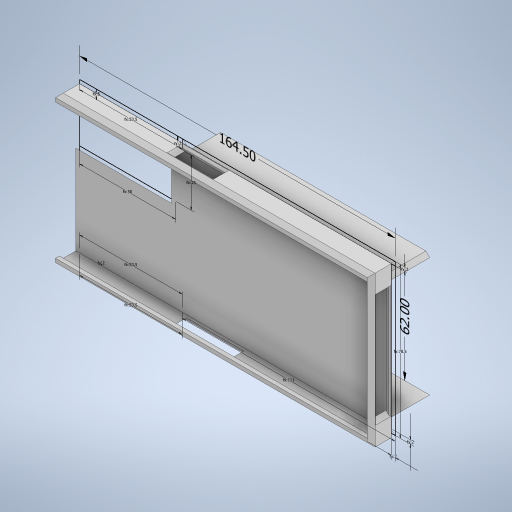
# Autodesk Inventor part: Case
Saved by Autodesk Inventor 2024 (Build 280153000, 153)
## iProperties
Created: 2024-07-02
Part Number: Case
Material: Generic
Document SubType Name: Modeling
Designer: Andrei
Density: 1 g/cm^3
Appearance: Default
Author: Andrei
Autodesk Inventor part; units mm, degrees
ref_plane "YZ Plane" through (0, 0, 0) normal (1, 0, 0) x (0, 1, 0)
ref_plane "XZ Plane" through (0, 0, 0) normal (0, 1, 0) x (-1, 0, 0)
ref_plane "XY Plane" through (0, 0, 0) normal (0, 0, 1) x (1, 0, 0)
sketch "Sketch1" plane through (0, 0, 0) normal (0, 0, 1) x (1, 0, 0)
  line L0 (-55.5, 39.25) -> (55.5, 39.25)
  line L1 (55.5, 39.25) -> (55.5, -39.25)
  line L2 (55.5, -39.25) -> (-55.5, -39.25)
  line L3 (-55.5, -39.25) -> (-55.5, 39.25)
  line L4 (-55.5, 39.25) -> (55.5, -39.25) construction
  line L5 (55.5, 39.25) -> (-55.5, -39.25) construction
  line L6 (-55.5, 39.25) -> (55.5, 39.25)
  line L7 (55.5, 39.25) -> (55.5, 37.25)
  line L8 (55.5, 37.25) -> (-55.5, 37.25)
  line L9 (-55.5, 37.25) -> (-55.5, 39.25)
  line L10 (55.5, 37.25) -> (53.5, 37.25)
  line L11 (53.5, 37.25) -> (53.5, -39.25)
  line L12 (53.5, -39.25) -> (55.5, -39.25)
  line L13 (55.5, -39.25) -> (55.5, 37.25)
  line L14 (-55.5, -39.25) -> (53.5, -39.25)
  line L15 (53.5, -39.25) -> (53.5, -37.25)
  line L16 (53.5, -37.25) -> (-55.5, -37.25)
  line L17 (-55.5, -37.25) -> (-55.5, -39.25)
  line L18 (-55.5, 39.25) -> (-109, 39.25)
  line L19 (-109, 39.25) -> (-109, -39.25)
  line L20 (-109, -39.25) -> (-55.5, -39.25)
  line L21 (-55.5, -39.25) -> (-55.5, 39.25)
  line L22 (-109, 34.25) -> (-59, 34.25)
  line L23 (-59, 34.25) -> (-59, 9.25)
  line L24 (-59, 9.25) -> (-109, 9.25)
  line L25 (-109, 9.25) -> (-109, 34.25)
  line L26 (-55.5, 39.25) -> (-109, 39.25)
  line L27 (-109, 39.25) -> (-109, 37.25)
  line L28 (-109, 37.25) -> (-55.5, 37.25)
  line L29 (-55.5, 37.25) -> (-55.5, 39.25)
  line L30 (-55.5, -39.25) -> (-109, -39.25)
  line L31 (-109, -39.25) -> (-109, -37.25)
  line L32 (-109, -37.25) -> (-55.5, -37.25)
  line L33 (-55.5, -37.25) -> (-55.5, -39.25)
  point P0 (0, 0)
  point P1 (-55.5, -37.25)
  point P2 (-55.5, 37.25)
  point P3 (-55.5, -37.25)
  dimension "d0" = 111
  dimension "d1" = 78.5
  dimension "d2" = 2
  dimension "d3" = 2
  dimension "d4" = 2
  dimension "d5" = 53.5
  dimension "d80" = 50
  dimension "d81" = 25
  dimension "d82" = 5
  dimension "d91" = 53.5
  dimension "d92" = 2
  dimension "d93" = 53.5
  dimension "d94" = 2
  constraints: 68 end point, 16 parallel, 8 horizontal, 8 perpendicular, 4 point on line, 2 midpoint
  measures "d0" distance of L1.end L2.end
  measures "d1" distance of L0.end L1.end
  measures "d2" distance of L6.end L7.end
  measures "d3" distance of L12.end L11.end
  measures "d4" distance of L15.end L14.end
  measures "d5" distance of L20.end L19.end
  measures "d80" distance of L23.end L24.end
  measures "d81" distance of L22.end L23.end
  measures "d82" distance between parallel lines of L18 L22
  measures "d91" distance of L28.end L27.end
  measures "d92" distance between parallel lines of L18 L28
  measures "d93" distance of L31.end L32.end
  measures "d94" distance between parallel lines of L30 L32
extrude "Extrusion1" add sketch "Sketch1" along normal blind 2 contours L8 L11 L16 L3
extrude "Extrusion2" add sketch "Sketch1" along normal blind 12.5 contours L0 L1 L8 L3 | L1 L2 L11 L8 | L16 L11 L2 L3
chamfer "Chamfer1" distance 2 angle 45 1 edges at (0, 39.25, 0)
chamfer "Chamfer2" distance 2 angle 45 1 edges at (55.5, -1, 0)
chamfer "Chamfer3" distance 2 angle 45 1 edges at (-1, -39.25, 0)
chamfer "Chamfer9" distance 2 angle 45 1 edges at (55.5, 0, 12.5)
extrude "Extrusion3" add sketch "Sketch1" along normal blind 2 contours L3 L28 L19 L18 | L3 L32 L19 L24 L23 L22 L28 | L3 L20 L19 L32 | L22 L23 L24 L19
chamfer "Chamfer13" distance 2 angle 45 1 edges at (-82.25, 39.25, 0)
chamfer "Chamfer14" distance 2 angle 45 1 edges at (-109, -1, 0)
chamfer "Chamfer15" distance 2 angle 45 1 edges at (-81.25, -39.25, 0)
sketch "Sketch2" plane through (0, 0, 0) normal (0, 0, -1) x (-1, 0, 0)
  line L0 (-53.5, 32) -> (53.5, 32)
  line L1 (53.5, 32) -> (53.5, -32)
  line L2 (53.5, -32) -> (-53.5, -32)
  line L3 (-53.5, -32) -> (-53.5, 32)
  line L4 (-53.5, 32) -> (53.5, -32) construction
  line L5 (53.5, 32) -> (-53.5, -32) construction
  line L6 (-53.5, -37.25) -> (-53.5, 37.25) projected
  line L7 (-53.5, 32) -> (57.5, 32)
  line L8 (57.5, 32) -> (57.5, 30)
  line L9 (57.5, 30) -> (-53.5, 30)
  line L10 (-53.5, 30) -> (-53.5, 32)
  line L11 (-53.5, -32) -> (55.5, -32)
  line L12 (55.5, -32) -> (55.5, -35.2285)
  line L13 (-53.5, -35.2285) -> (-53.5, -32)
  line L14 (-53.5, -32) -> (57.5, -32)
  line L15 (57.5, -32) -> (57.5, -34)
  line L16 (57.5, -34) -> (-53.5, -34)
  line L17 (-53.5, -34) -> (-53.5, -32)
  line L18 (57.5, 30) -> (61.5, 30)
  line L19 (61.5, -32) -> (59.5, -32)
  line L20 (57.5, 30) -> (55.5, 30)
  line L21 (55.5, 30) -> (55.5, -32)
  line L22 (55.5, -32) -> (57.5, -32)
  line L23 (57.5, -32) -> (57.5, 30)
  point P0 (0, 0)
  point P1 (55.5, 30)
  point P2 (-53.5, -32)
  dimension "d57" = 107
  dimension "d58" = 64
  dimension "d59" = 111
  dimension "d60" = 2
  dimension "d61" = 109
  dimension "d62" = 111
  dimension "d63" = 2
  dimension "d64" = 2
  dimension "d65" = 2
  constraints: 46 end point, 10 parallel, 7 point on line, 6 horizontal, 5 perpendicular, 2 midpoint
  measures "d57" distance of L0.start L0.end
  measures "d58" distance of L0.end L1.end
  measures "d59" distance of L8.end L9.end
  measures "d60" distance of L7.end L8.end
  measures "d61" distance of L12.end L13.start
  measures "d62" distance of L15.end L16.end
  measures "d63" distance between parallel lines of L16 L14
  measures "d64" distance of L19.start L19.end
  measures "d65" distance of L22.end L21.end
extrude "Extrusion4" add sketch "Sketch2" along normal blind 20 contours L0 L1 L9 L3 | L7 L8 L9 L1 | L2 L11 L12 L16 L6 | L9 L23 L14 L21 | L14 L15 L16 L12
chamfer "Chamfer16" distance 2 angle 45 4 edges at (-57.5, -34, -10) (-57.5, 32, -10) (53.5, 32, -10) (53.5, -34, -10)
sketch "Sketch3" plane through (-57.5, -32, 0) normal (-1, 0, 0) x (0, 0, 1)
  line L0 (0, 0) -> (-20, 0) projected
  line L1 (0, 62) -> (-20, 62) projected
  line L2 (-20, 0) -> (0, 62)
  line L3 (-20, 62) -> (-20, 64) projected
  line L4 (-20, 62) -> (0, 0)
  circle A0 centre (-10, 31) radius 2.5
  point P0 (0, 32)
  dimension "d71" = 5
  constraints: 4 end point, 1 centre point, 1 midpoint
  measures "d71" diameter of A0
hole "Hole1" at (-57.5, -1, -10) direction (1, 0, 0) diameter 9.2964 end through all counterbore diameter 9.525 counterbore depth 5
extrude "Extrusion5" cut sketch "Sketch1" along normal blind 10 contours L22 L23 L24 L19
chamfer "Chamfer17" distance 1 angle 45 1 edges at (-59, 21.75, 0)
chamfer "Chamfer18" distance 2 angle 45 4 edges at (-58.5, 34.25, 0) (-83.0001, 34.25, 0) (-58.5, 9.25, 0) (-83.0001, 9.25, 0)
extrude "Extrusion6" add sketch "Sketch1" along normal blind 12.5 contours L3 L28 L19 L18 | L3 L20 L19 L32
chamfer "Chamfer19" distance 2 angle 45 6 edges at (-27.7499, -39.25, 12.5) (-27.75, 39.25, 12.5) (-109, -39.25, 6.25) (-109, 39.25, 6.25) (-82.25, 39.25, 0) (-82.25, -39.25, 0)
sketch "Sketch4" plane through (55.5, -39.25, 2) normal (1, 0, 0) x (0, 0, -1)
  line L0 (0, 0) -> (-8.5, 0) projected
  line L1 (0, 78.5) -> (0, 0) projected
  line L2 (-8.5, 0) -> (0, 78.5)
  line L3 (-8.5, 0) -> (-8.5, 78.5) projected
  line L4 (-8.5, 78.5) -> (0, 0)
  line L5 (-7.75, 11.75) -> (-0.75, 11.75)
  line L6 (-0.75, 11.75) -> (-0.75, 66.75)
  line L7 (-0.75, 66.75) -> (-7.75, 66.75)
  line L8 (-7.75, 66.75) -> (-7.75, 11.75)
  line L9 (-7.75, 11.75) -> (-0.75, 66.75) construction
  line L10 (-0.75, 11.75) -> (-7.75, 66.75) construction
  point P0 (2, 39.25)
  point P1 (-4.25, 39.25)
  dimension "d100" = 7
  dimension "d101" = 55
  constraints: 16 end point, 3 midpoint, 2 parallel, 1 horizontal, 1 perpendicular
  measures "d100" distance of L7.end L6.end
  measures "d101" distance of L6.end L5.end
extrude "Extrusion7" cut sketch "Sketch4" against normal blind 10 contours L5 L2 L4 | L4 L2 L7 L6 L5 | L5 L8 L7 L4 L2 | L2 L4 L7
chamfer "Chamfer20" distance 2 angle 45 2 edges at (55.5, -27.5, 6.25) (55.5, 27.5, 6.25)
chamfer "Chamfer21" distance 0.5 angle 45 6 edges at (55.5, -28.4999, 9.75) (55.5, 0, 9.75) (55.5, 28.4999, 9.75) (55.5, -28.5, 2.75) (55.5, 0, 2.75) (55.5, 28.4999, 2.75)
sketch "Sketch5" plane through (-107, 39.25, 2) normal (0, 1, 0) x (1, 0, 0)
  line L0 (76, -7.25) -> (56, -7.25)
  line L1 (56, -7.25) -> (56, -1.25)
  line L2 (56, -1.25) -> (76, -1.25)
  line L3 (76, -1.25) -> (76, -7.25)
  line L4 (-2, 0) -> (-2, -10.5) projected
  line L5 (162.5, -8.5) -> (0, -8.5) projected
  point P0 (107, 2)
  point P1 (56, -4.25)
  point P2 (-2, -5.25)
  dimension "d110" = 20
  dimension "d111" = 6
  dimension "d112" = 58
  dimension "d115" = 4.25
  constraints: 8 end point, 2 midpoint, 2 parallel, 1 horizontal, 1 perpendicular
  measures "d110" distance of L1.end L2.end
  measures "d111" distance of L0.end L1.end
  measures "d112" horizontal distance of point (56, -4.25) point (-2, -5.25)
  measures "d115" distance from line of L5 point (56, -4.25)
extrude "Extrusion8" cut sketch "Sketch5" along normal mid plane 10
chamfer "Chamfer22" distance 2 angle 45 2 edges at (-31, 39.25, 6.25) (-51, 39.25, 6.25)
chamfer "Chamfer23" distance 1 angle 45 6 edges at (-30.0001, 39.25, 9.25) (-41, 39.25, 9.25) (-52, 39.25, 9.25) (-30.0001, 39.25, 3.25) (-41, 39.25, 3.25) (-52, 39.25, 3.25)
sketch "Sketch6" plane through (-107, -39.25, 2) normal (0, -1, 0) x (1, 0, 0)
  line L0 (87, 1.25) -> (57, 1.25)
  line L1 (57, 1.25) -> (57, 7.25)
  line L2 (57, 7.25) -> (87, 7.25)
  line L3 (87, 7.25) -> (87, 1.25)
  line L4 (162.5, 0) -> (0, 0) projected
  line L5 (-2, 0) -> (-2, 10.5) projected
  point P0 (107, -2)
  point P1 (57, 4.25)
  dimension "d122" = 30
  dimension "d123" = 6
  dimension "d124" = 1.25
  dimension "d125" = 59
  constraints: 8 end point, 2 parallel, 1 horizontal, 1 midpoint, 1 perpendicular
  measures "d122" distance of L1.end L2.end
  measures "d123" distance of L0.end L1.end
  measures "d124" distance between parallel lines of L4 L0
  measures "d125" distance from line of point (57, 4.25) L5
extrude "Extrusion9" cut sketch "Sketch6" along normal mid plane 10
chamfer "Chamfer24" distance 2 angle 45 2 edges at (-50, -39.25, 6.25) (-20, -39.25, 6.25)
chamfer "Chamfer25" distance 1 angle 45 6 edges at (-50.9999, -39.25, 3.25) (-35, -39.25, 3.25) (-19.0001, -39.25, 3.25) (-50.9999, -39.25, 9.25) (-35, -39.25, 9.25) (-19.0001, -39.25, 9.25)
sketch "Sketch7" plane through (-109, -37.25, 2) normal (0, 1, 0) x (1, 0, 0)
  line L0 (162.5, -10.5) -> (0, -10.5) projected
  line L1 (162.5, 0) -> (162.5, -10.5) projected
  line L2 (0, -10.5) -> (162.5, -10.5)
  line L3 (162.5, -10.5) -> (162.5, -8.5)
  line L4 (162.5, -8.5) -> (0, -8.5)
  line L5 (0, -8.5) -> (0, -10.5)
  point P0 (109, 2)
  dimension "d137" = 2
  constraints: 8 end point, 2 parallel, 1 horizontal, 1 perpendicular, 1 point on line
  measures "d137" distance of L3.end L2.end
extrude "Extrusion10" add sketch "Sketch7" along normal blind 2
sketch "Sketch8" plane through (-109, 37.25, 2) normal (0, -1, 0) x (1, 0, 0)
  line L0 (0, 10.5) -> (162.5, 10.5) projected
  line L1 (0, 10.5) -> (162.5, 10.5)
  line L2 (162.5, 10.5) -> (162.5, 8.5)
  line L3 (162.5, 8.5) -> (0, 8.5)
  line L4 (0, 8.5) -> (0, 10.5)
  point P0 (109, -2)
  dimension "d140" = 162.5
  dimension "d141" = 2
  constraints: 8 end point, 2 parallel, 1 horizontal, 1 perpendicular
  measures "d140" distance of L2.end L3.end
  measures "d141" distance of L1.end L2.end
extrude "Extrusion11" add sketch "Sketch8" along normal blind 2
equation "\"d0\" = fluovisorHeight + 2 * wallThickness"
equation "\"d1\" = smartphoneWidth + 2 * wallThickness"
equation "\"d2\" = wallThickness"
equation "\"d3\" = wallThickness"
equation "\"d4\" = wallThickness"
equation "\"d5\" = 0.5 * fluovisorHeight"
equation "\"d80\" = camerasHeight"
equation "\"d81\" = camerasWidth"
equation "\"d82\" = dist2cameras"
equation "\"d91\" = 0.5 * fluovisorHeight"
equation "\"d92\" = wallThickness"
equation "\"d93\" = 0.5 * fluovisorHeight"
equation "\"d94\" = wallThickness"
equation "\"d6\" = wallThickness"
equation "\"d8\" = 2 * wallThickness + smartphoneDepth"
equation "\"d40\" = wallThickness"
equation "\"d57\" = lAkkum"
equation "\"d59\" = lAkkum + 2 * wallThickness"
equation "\"d60\" = wallThickness"
equation "\"d61\" = lAkkum + wallThickness"
equation "\"d62\" = lAkkum + 2 * wallThickness"
equation "\"d63\" = wallThickness"
equation "\"d64\" = wallThickness"
equation "\"d65\" = wallThickness"
equation "\"d95\" = 2 * wallThickness + smartphoneDepth"
equation "\"d110\" = powerOnButtonWidth"
equation "\"d111\" = powerOnButtonHeight"
equation "\"d115\" = 0.5 * smartphoneDepth"
equation "\"d122\" = volumeButtonsWidth"
equation "\"d123\" = volumeButtonsHeight"
equation "\"d124\" = 0.5 * smartphoneDepth - 0.5 * volumeButtonsHeight"
equation "\"d137\" = wallThickness"
equation "\"d138\" = wallThickness"
equation "\"d141\" = wallThickness"
equation "\"d142\" = wallThickness"
equation "\"smartphoneWidth\" = 74.5"
equation "\"smartphoneDepth\" = 8.5"
equation "\"fluovisorHeight\" = 107"
equation "\"wallThickness\" = 2"
equation "\"holesDistance\" = 1"
equation "\"dHoles\" = 3"
equation "\"lAkkum\" = 107"
equation "\"hAkkum\" = 6"
equation "\"camerasWidth\" = 25"
equation "\"camerasHeight\" = 50"
equation "\"dist2cameras\" = 5"
equation "\"powerOnButtonHeight\" = 6"
equation "\"powerOnButtonWidth\" = 20"
equation "\"volumeButtonsWidth\" = 30"
equation "\"volumeButtonsHeight\" = 6"
body "Solid1"
